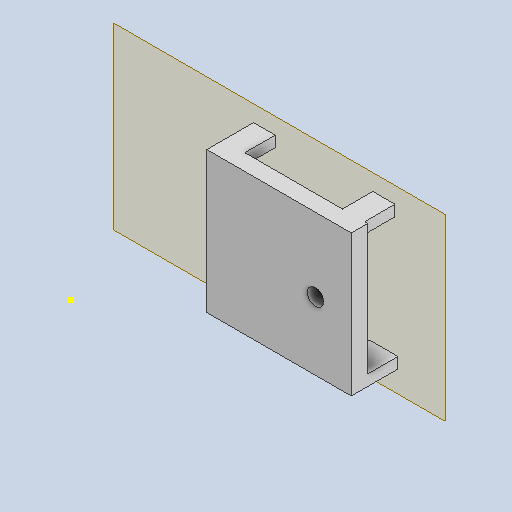
# Autodesk Inventor part: 0904-idler-supporter
Saved by Autodesk Inventor 2024.3 (Build 283343000, 343)
## iProperties
Created: 2024-09-04
Part Number: 0904-idler-supporter
Material: 일반
Document SubType Name: Modeling
Designer: gretc
Density: 1 g/cm^3
Appearance: 기본값
Author: gretc
Autodesk Inventor part; units mm, degrees
ref_plane "YZ Plane" through (0, 0, 0) normal (1, 0, 0) x (0, 1, 0)
ref_plane "XZ Plane" through (0, 0, 0) normal (0, 1, 0) x (-1, 0, 0)
ref_plane "XY Plane" through (0, 0, 0) normal (0, 0, 1) x (1, 0, 0)
ref_plane "작업 평면1" through (0, 0, 0) normal (0, 0, 1) x (1, 0, 0)
sketch "스케치1" plane through (0, 0, 0) normal (0, 0, 1) x (1, 0, 0)
  line L0 (8, 36.5) -> (2, 36.5) projected
  line L1 (2, 36.5) -> (2, 10.5) projected
  line L2 (4.8997, 10.5) -> (2, 10.5) projected
  line L3 (5.1003, 10.5) -> (4.8997, 10.5) projected
  line L4 (8.5, 10.5) -> (5.1003, 10.5) projected
  line L5 (8.5, 24) -> (8.5, 10.5) projected
  line L6 (8.5, 24) -> (11.05, 24) projected
  line L7 (11.05, 24) -> (11.05, 25.4) projected
  line L8 (9.6, 25.4) -> (11.05, 25.4) projected
  line L9 (9.6, 25.4) -> (9.6, 35.5) projected
  line L10 (9.6, 35.5) -> (22.4, 35.5) projected
  line L11 (22.4, 25.4) -> (22.4, 35.5) projected
  line L12 (20.95, 25.4) -> (22.4, 25.4) projected
  line L13 (20.95, 24) -> (20.95, 25.4) projected
  line L14 (20.95, 24) -> (23.5, 24) projected
  line L15 (23.5, 24) -> (23.5, 19.4) projected
  line L16 (23.5, 19.4) -> (24.7124, 19.4) projected
  line L17 (24.7124, 10.5) -> (24.7124, 19.4) projected
  line L18 (26.8997, 10.5) -> (24.7124, 10.5) projected
  line L19 (27.1003, 10.5) -> (26.8997, 10.5) projected
  line L20 (30.975, 10.5) -> (27.1003, 10.5) projected
  line L21 (30.975, 10.5) -> (30.975, 8) projected
  line L22 (30.975, 8) -> (45.025, 8) projected
  line L23 (45.025, 10.5) -> (45.025, 8) projected
  line L24 (48.8997, 10.5) -> (45.025, 10.5) projected
  line L25 (49.1003, 10.5) -> (48.8997, 10.5) projected
  line L26 (52.975, 10.5) -> (49.1003, 10.5) projected
  line L27 (52.975, 10.5) -> (52.975, 8) projected
  line L28 (52.975, 8) -> (57.5, 8) projected
  line L29 (57.5, 38) -> (57.5, 8) projected
  line L30 (52, 38) -> (57.5, 38) projected
  line L31 (52, 36.5) -> (52, 38) projected
  line L32 (52, 36.5) -> (46, 36.5) projected
  line L33 (46, 38) -> (46, 36.5) projected
  line L34 (30, 38) -> (46, 38) projected
  line L35 (30, 36.5) -> (30, 38) projected
  line L36 (30, 36.5) -> (24, 36.5) projected
  line L37 (24, 38) -> (24, 36.5) projected
  line L38 (8, 38) -> (24, 38) projected
  line L39 (8, 36.5) -> (8, 38) projected
  line L40 (24.9998, 36.5) -> (28.9963, 36.5)
  line L41 (28.9963, 36.5) -> (28.9963, 34.5)
  line L42 (28.9963, 34.5) -> (24.9998, 34.5)
  line L43 (24.9998, 34.5) -> (24.9998, 36.5)
  line L44 (46.9624, 36.5) -> (51.0376, 36.5)
  line L45 (51.0376, 36.5) -> (51.0376, 34.5)
  line L46 (51.0376, 34.5) -> (46.9624, 34.5)
  line L47 (46.9624, 34.5) -> (46.9624, 36.5)
  line L48 (29.5978, 10.5) -> (24.7124, 10.5)
  line L49 (24.7124, 10.5) -> (24.7124, 12.5)
  line L50 (24.7124, 12.5) -> (29.5978, 12.5)
  line L51 (29.5978, 12.5) -> (29.5978, 10.5)
  line L52 (46.2621, 10.5) -> (51.5945, 10.5)
  line L53 (51.5945, 10.5) -> (51.5945, 12.5)
  line L54 (51.5945, 12.5) -> (46.2621, 12.5)
  line L55 (46.2621, 12.5) -> (46.2621, 10.5)
  line L56 (44.9509, 9.2001) -> (71.1438, 9.107) projected
  line L57 (71.2419, 36.7068) -> (45.0491, 36.7999) projected
  point P0 (0, 0)
  point P1 (46.9624, 35.5)
  point P2 (51.0376, 35.5)
  point P3 (46.2621, 11.5)
  point P4 (51.5945, 11.5)
  point P5 (24.7124, 11.5)
  point P6 (29.5978, 11.5)
  point P7 (24.9998, 35.5)
  point P8 (28.9963, 35.5)
  dimension "d0" = 2
  dimension "d1" = 2
  dimension "d2" = 2
  dimension "d3" = 2
  dimension "d4" = 4.0753
  dimension "d5" = 5.3324
  dimension "d6" = 6.4624
  dimension "d7" = 5.9055
  dimension "d8" = 4.8853
  dimension "d9" = 3.9966
  dimension "d10" = 2.5998
  constraints: 32 end point, 8 midpoint, 8 parallel, 7 point on line, 4 perpendicular, 1 collinear
  measures "d0" distance of L40.end L41.end
  measures "d1" distance of L44.end L45.end
  measures "d2" distance of L17.start L49.end
  measures "d3" distance of L53.end L52.end
  measures "d4" distance of point (46.962, 35.5) point (51.038, 35.5)
  measures "d5" distance of point (46.262, 11.5) point (51.594, 11.5)
  measures "d6" distance between parallel lines of L45 L29
  measures "d7" distance between parallel lines of L53 L29
  measures "d8" distance of point (24.712, 11.5) point (29.598, 11.5)
  measures "d9" distance of point (25, 35.5) point (28.996, 35.5)
  measures "d10" distance between parallel lines of L11 L43
extrude "돌출1" add sketch "스케치1" along normal blind 5.6 contours L36 L41 L42 L43 | L32 L45 L46 L47 | L26 L25 L24 L55 L54 L53 | L50 L51 L20 L19 L18 L17
sketch "스케치2" plane through (0, 0, 5.6) normal (0, 0, 1) x (1, 0, 0)
  line L0 (46.2621, 12.5) -> (46.2621, 10.5) projected
  line L1 (46.2621, 10.5) -> (51.5945, 10.5) projected
  line L2 (51.5945, 10.5) -> (51.5945, 12.5) projected
  line L3 (51.5945, 12.5) -> (46.2621, 12.5) projected
  line L4 (29.5978, 12.5) -> (24.7124, 12.5) projected
  line L5 (24.7124, 12.5) -> (24.7124, 10.5) projected
  line L6 (24.7124, 10.5) -> (29.5978, 10.5) projected
  line L7 (29.5978, 10.5) -> (29.5978, 12.5) projected
  line L8 (28.9963, 34.5) -> (28.9963, 36.5) projected
  line L9 (28.9963, 36.5) -> (24.9998, 36.5) projected
  line L10 (24.9998, 36.5) -> (24.9998, 34.5) projected
  line L11 (24.9998, 34.5) -> (28.9963, 34.5) projected
  line L12 (51.0376, 34.5) -> (51.0376, 36.5) projected
  line L13 (51.0376, 36.5) -> (46.9624, 36.5) projected
  line L14 (46.9624, 36.5) -> (46.9624, 34.5) projected
  line L15 (46.9624, 34.5) -> (51.0376, 34.5) projected
  line L16 (51.5945, 10.5) -> (24.9998, 10.5)
  line L17 (24.9998, 10.5) -> (24.9998, 36.5)
  line L18 (24.9998, 36.5) -> (51.5945, 36.5)
  line L19 (51.5945, 36.5) -> (51.5945, 10.5)
  point P0 (0, 0)
  constraints: 8 end point, 2 parallel, 1 horizontal, 1 perpendicular
extrude "돌출2" add sketch "스케치2" along normal blind 3 contours L3 L2 L1 L0 | L0 L16 L7 L4 L17 L11 L8 L18 L14 L15 L12 L19 L3 | L6 L17 L4 L7 | L12 L15 L14 L13 | L10 L9 L8 L11
sketch "스케치3" plane through (0, 0, 8.6) normal (0, 0, 1) x (1, 0, 0)
  point P0 (0, 0)
sketch "스케치4" plane through (0, 0, 8.6) normal (0, 0, 1) x (1, 0, 0)
  circle A0 centre (45, 23) radius 1.5 projected
  circle A1 centre (45, 23) radius 13.9 projected
  circle A2 centre (52.7782, 30.7782) radius 1.25 projected
  line L0 (56, 10) -> (56, 36) projected
  circle A3 centre (55.9999, 22.9609) radius 1.2812 projected
  circle A4 centre (52.7782, 15.2218) radius 1.55 projected
  circle A5 centre (45, 12) radius 1.55 projected
  circle A6 centre (37.2218, 15.2218) radius 1.55 projected
  circle A7 centre (34, 23) radius 1.55 projected
  circle A8 centre (37.2495, 30.8058) radius 1.2812 projected
  circle A9 centre (45, 34) radius 1.55 projected
  point P0 (0, 0)
extrude "돌출3" cut sketch "스케치4" against normal blind 3 contours A0
